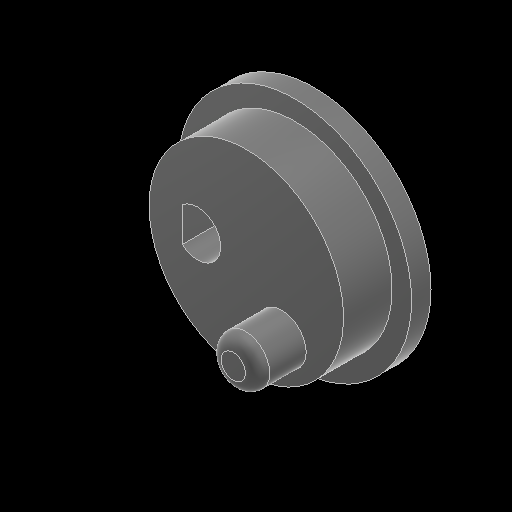
# Autodesk Inventor part: ShufflerBaseCam
Saved by Autodesk Inventor 2023 (Build 270158000, 158)
## iProperties
Created: 2022-03-05
Part Number: ShufflerBaseCam
Material: Nylon 6
Document SubType Name: Modeling
Designer: tandu
Density: 1.12 g/cm^3
Appearance: Smooth - Black
Mass: 1.61207 g
Surface Area: 11.5584 cm^2
Volume: 1.33229 cm^3
CamSize1: 0.50000000 in
NubAngle1: 30.00000000 deg
Offset1: 0.12500000 in
Author: tandu
Autodesk Inventor part; units mm, degrees
ref_plane "YZ Plane" through (0, 0, 0) normal (1, 0, 0) x (0, 1, 0)
ref_plane "XZ Plane" through (0, 0, 0) normal (0, 1, 0) x (-1, 0, 0)
ref_plane "XY Plane" through (0, 0, 0) normal (0, 0, 1) x (1, 0, 0)
sketch "Sketch1" plane through (0, 0, 0) normal (0, 0, 1) x (1, 0, 0)
  line L0 (23.8099, -26.8968) -> (23.8099, -29.4948)
  line L1 (23.8099, -29.4948) -> (21.5599, -30.7939)
  line L2 (21.5599, -30.7939) -> (19.3099, -29.4948)
  line L3 (19.3099, -29.4948) -> (19.3099, -26.8968)
  line L4 (19.3099, -26.8968) -> (21.5599, -25.5977)
  line L5 (21.5599, -25.5977) -> (23.8099, -26.8968)
  line L6 (2.25, 1.299) -> (2.25, -1.299) construction
  line L7 (2.25, -1.299) -> (0, -2.5981) construction
  line L8 (0, -2.5981) -> (-2.25, -1.299) construction
  line L9 (-2.25, -1.299) -> (-2.25, 1.299) construction
  line L10 (-2.25, 1.299) -> (0, 2.5981) construction
  line L11 (0, 2.5981) -> (2.25, 1.299) construction
  line L12 (2.25, -1.299) -> (-2.25, 1.299) construction
  line L13 (-2.25, -1.299) -> (2.25, 1.299) construction
  line L14 (0, 2.5981) -> (0, -2.5981) construction
  circle A0 centre (3.175, 0) radius 6.35
  circle A1 centre (3.175, 0) radius 7.62
  circle A2 centre (0, 0) radius 1.5
  line L15 (-1, 1.118) -> (-1, -1.118)
  dimension "d2" = 60
  dimension "d3" = 4.5
  dimension "d4" = 60
  dimension "d5" = 4.5
  dimension "d6" = 12.7
  dimension "d7" = 3.175
  dimension "d8" = 1.27
  dimension "d19" = 3
  dimension "d20" = 2.2361
  constraints: 32 end point, 10 equal length, 5 horizontal alignment, 4 parallel, 4 vertical, 3 centre point, 2 coincident, 2 point on circle, 2 vertical alignment, 1 midpoint
  measures "d2" angle of L0 L5
  measures "d3" distance between parallel lines of L3 L0
  measures "d4" angle of L6 L11
  measures "d5" distance between parallel lines of L9 L6
  measures "d6" diameter of A0
  measures "d7" distance of point (0, 0) A0.centre
  measures "d8" radial gap between concentric circles of A0 A1
  measures "d19" diameter of A2
  measures "d20" distance of L15.start L15.end
extrude "Lip" add sketch "Sketch1" along normal blind 1.27 contours A0 | A1 | L15 A2 picked at (-1.1631, -0.0599)
extrude "Cam" add sketch "Sketch1" along normal blind 3.175 from surface at 1.27 contours A0 | L15 A2 picked at (-1.1631, -0.0599)
sketch "Sketch2" plane through (3.175, 0, 4.445) normal (0, 0, 1) x (1, 0, 0)
  circle A0 centre (2.3243, -3.175) radius 1.5875
  line L0 (-3.175, 0) -> (5.1771, 0) construction
  line L1 (-3.175, 0) -> (2.3243, -3.175) construction
  dimension "d13" = 3.175
  dimension "d14" = 30
  dimension "d15" = 6.35
  constraints: 4 end point, 1 centre point, 1 horizontal
  measures "d13" diameter of A0
  measures "d14" angle of L1 L0
  measures "d15" distance of L0.start L1.end
extrude "Nub" add sketch "Sketch2" along normal blind 3.175
fillet "Fillet1" radius 0.7937 1 edges at (3.9118, -3.175, 7.62)
equation "\"d5\" = HexSize"
equation "\"d6\" = CamSize1"
equation "\"d7\" = Offset1"
equation "\"d11\" = FootThickness"
equation "\"d13\" = FootThickness"
equation "\"d14\" = NubAngle1"
equation "\"d15\" = NubOffset"
equation "\"d16\" = FootThickness"
equation "\"Offset1\" = Offset"
equation "\"NubAngle1\" = NubAngle"
equation "\"CamSize1\" = CamSize"
equation "\"HexSize\" = 4.5"
equation "\"FootThickness\" = 3.175"
equation "\"NubOffset\" = 6.35"
equation "\"Offset\" = 3.175"
equation "\"NubAngle\" = 30deg"
equation "\"CamSize\" = 12.7"
body "Solid1"
